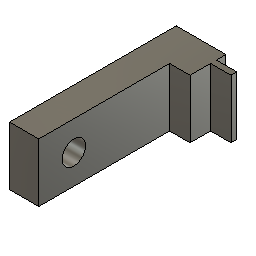
İmkansızlar Birleştirme Parçası v15 (Autodesk Fusion 360 design; units mm, degrees)
Autodesk Fusion 360 part; units mm, degrees
note: some values were not read from the file. Set by a fixed rule: which sketch regions a step uses.
sketch "Eskiz1" plane through (0, 0, 0) normal (0, 1, 0) x (1, 0, 0)
  line L0 (0, -11.5) -> (0, 0)
  line L1 (0, 0) -> (15, 0)
  line L2 (15, 0) -> (15, -45)
  line L3 (15, -45) -> (0, -45)
  line L4 (0, -45) -> (0, 0)
  dimension "d3" = 15
  dimension "d4" = 45
  constraint vertical L0
  constraint coincident L0.end L1.start
  constraint horizontal L1
  constraint vertical L2
  constraint horizontal L3
  constraint vertical L4
  measures "d3" distance of L0.end L1.end
  measures "d4" distance of L0.end L3.end
extrude "Ekstrüde Et1" add sketch "Eskiz1" along normal blind 20
sketch "Eskiz2" plane through (0, 0, 0) normal (-1, 0, 0) x (0, 0, 1)
  line L0 (0, 0) -> (45, 0)
  line L1 (45, 0) -> (45, 20)
  line L2 (45, 20) -> (0, 20)
  line L3 (0, 20) -> (0, 0)
  line L4 (0, 0) -> (15, 0)
  line L5 (15, 0) -> (15, 20)
  line L6 (15, 20) -> (0, 20)
  line L7 (0, 20) -> (0, 0)
  circle A0 centre (33, 10) radius 4
  point P0 (37, 10)
  dimension "d7" = 15
  dimension "d8" = 20
  dimension "d9" = 8
  dimension "d10" = 8
  constraint horizontal L4
  constraint vertical L5
  constraint horizontal L6
  constraint vertical L7
  constraint coincident L0.start L3.end
  constraint coincident A0 P0
  measures "d7" distance of L0.start L4.end
  measures "d8" distance of L0.start L2.end
  measures "d9" diameter of A0
  measures "d10" distance of L1 P0
extrude "Ekstrüde Et2" cut sketch "Eskiz2" against normal blind 20 contours A0
sketch "Eskiz4" plane through (15, 0, 0) normal (1, 0, 0) x (0, 0, -1)
  circle A0 centre (-33, 10) radius 4
  line L0 (-45, 0) -> (0, 0)
  line L1 (0, 0) -> (0, 20)
  line L2 (0, 20) -> (-45, 20)
  line L3 (-45, 20) -> (-45, 0)
  line L4 (0, 0) -> (-10, 0)
  line L5 (-10, 0) -> (-10, 20)
  line L6 (-10, 20) -> (0, 20)
  line L7 (0, 20) -> (0, 0)
  dimension "d22" = 10
  constraint horizontal L4
  constraint vertical L5
  constraint horizontal L6
  constraint vertical L7
  constraint coincident L0.end L1.start
  measures "d22" distance of L0.end L4.end
extrude "Ekstrüde Et6" add sketch "Eskiz4" along normal blind 7 contours L0 L1 L2 L4 L5 L6 L7
sketch "Eskiz5" plane through (0, 0, 0) normal (0, 0, -1) x (-1, 0, 0)
  line L0 (-22, 0) -> (0, 0)
  line L1 (0, 0) -> (0, 20)
  line L2 (0, 20) -> (-22, 20)
  line L3 (-22, 20) -> (-22, 0)
  line L4 (-22, 0) -> (-15, 0)
  line L5 (-15, 0) -> (-15, 20)
  line L6 (-15, 20) -> (-22, 20)
  line L7 (-22, 20) -> (-22, 0)
  dimension "d25" = 7
  dimension "d26" = 20
  constraint horizontal L4
  constraint vertical L5
  constraint horizontal L6
  constraint vertical L7
  constraint coincident L0.start L3.end
  measures "d25" distance of L0.start L4.end
  measures "d26" distance of L0.start L2.end
extrude "Ekstrüde Et7" add sketch "Eskiz5" along normal blind 12 contours L0 L2 L3 L4 L5 L6 L7
extrude "Ekstrüde Et9" cut 1 faces at (0, 10, 9.6667) along direction (1, 0, 0) blind 5
sketch "Eskiz7" plane through (22, 0, 0) normal (1, 0, 0) x (0, 0, -1)
  line L0 (12, 20) -> (-10, 20)
  line L1 (-10, 20) -> (-10, 0)
  line L2 (-10, 0) -> (12, 0)
  line L3 (12, 0) -> (12, 20)
  line L4 (6.7308, 20) -> (8.7308, 20)
  line L5 (8.7308, 20) -> (8.7308, 0)
  line L6 (8.7308, 0) -> (6.7308, 0)
  line L7 (6.7308, 0) -> (6.7308, 20)
  dimension "d36" = 2
  constraint horizontal L4
  constraint vertical L5
  constraint horizontal L6
  constraint vertical L7
  constraint coincident L0 L4.start
  measures "d36" distance of L4.start L4.end
extrude "Ekstrüde Et10" add sketch "Eskiz7" along normal blind 7 contours L0 L2 L4 L5 L6 L7
extrude "Ekstrüde Et11" add 1 faces at (11.6667, 13.3333, 0) along direction (0, 0, -1) blind 12
extrude "Ekstrüde Et12" cut 1 faces at (17.3333, 6.6667, 10) along direction (0, 0, -1) blind 9.731
